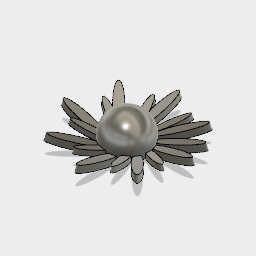
花 v0 (Autodesk Fusion 360 design; units mm, degrees)
Autodesk Fusion 360 part; units mm, degrees
sketch "草图1" plane through (0, 0, 0) normal (0, 1, 0) x (1, 0, 0)
  ellipse E0 centre (0, 0) end of major axis (0, 10) minor radius 2
  line L0 (0, -10) -> (0, 10)
  line L1 (2, 0) -> (-2, 0)
extrude "拉伸1" add sketch "草图1" along normal blind 3 makes body 1
move_body "移动1" bodies 1 to x (1, 0, 0) y (0, 0.965926, 0.258819) z (0, -0.258819, 0.965926) at (0, -0.2218, -0.4814)
box "长方体基本要素1" add length 2 width 2 height 2 placed x (0, 0, 1) y (1, 0, 0) z (0, 1, 0) at (1, 0, 17) separate body makes body 2
pattern_circular "C-阵列1" count 8 over 360 about axis through (3, 2, 17) along (0, -1, 0) of bodies 1 makes body 3 at (15.365, 0.4232, 1.2382) makes body 4 at (22.8886, 0.4232, 14.5981) makes body 5 at (18.7618, 0.4232, 29.365) makes body 6 at (5.4019, 0.4232, 36.8886) makes body 7 at (-8.8159, 3.321, 32.2127) makes body 8 at (-12.0742, -0.8668, 20.5981) makes body 9 at (-12.7618, 0.4232, 4.635)
copy_body "复制和粘贴实体1" bodies 4 1 8 3 5 7 9 6 makes body 10 makes body 11 makes body 12 makes body 13 makes body 14 makes body 15 makes body 16 makes body 17
scale "缩放1" factor 0.8 about (5.8608, 0.0878, 9.8966) bodies 14 12 15 10 11 17 16
move_body "移动2" bodies 13 10 14 17 15 12 16 11 2 to x (0.906308, 0, 0.422618) y (0, 1, 0) z (-0.422618, 0, 0.906308) at (7.4656, 0, 0.3249)
sphere "球体基本要素2" add diameter 20 placed x (1, 0, 0) y (0, 0, -1) z (0, 1, 0) at (-34, 0, 43) separate body makes body 18
move_body "MoveFace1" bodies 18 to x (1, 0, 0) y (0, 1, 0) z (0, 0, 1) at (37.1063, 2.9844, -25.4671) on bodies 18
combine "合并1" operation add target body 18 tool bodies 4 13 3 11 1 16 9 12 8 15 7 17 6 14 5 10
box "长方体基本要素2" add length 22 width 45 height 10 placed x (0, 0, -1) y (-1, 0, 0) z (0, 1, 0) at (45, 0, 77) separate body makes body 19
move_body "移动3" bodies 19 to x (1, 0, 0) y (0, 1, 0) z (0, 0, 1) at (-18.205, -12.9325, -48.6461)
combine "合并2" operation cut target body 18 tool bodies 19
sphereprimitive "球体基本要素1" [rolled back] diameter 20
hidden bodies 2
